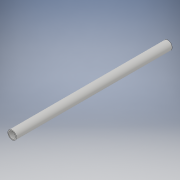
# Autodesk Inventor part: Prop Rod
Saved by Autodesk Inventor 2019 (Build 230136000, 136)
## iProperties
Created: 2019-10-06
Part Number: Prop Rod
Material: Generic
Document SubType Name: Modeling
Designer: robgr
Density: 1 g/cm^3
Appearance: Default
Author: robgr
Autodesk Inventor part; units mm, degrees
ref_plane "YZ Plane" through (0, 0, 0) normal (1, 0, 0) x (0, 1, 0)
ref_plane "XZ Plane" through (0, 0, 0) normal (0, 1, 0) x (-1, 0, 0)
sketch "Sketch1" plane through (0, 0, 0) normal (0, 0, 1) x (1, 0, 0)
  circle A0 centre (0, 0) radius 7.5
  circle A1 centre (0, 0) radius 6
  dimension "d0" = 15
  dimension "d1" = 12
  constraints: 2 centre point, 2 coincident
  measures "d0" diameter of A0
  measures "d1" diameter of A1
extrude "Extrusion1" add sketch "Sketch1" along normal blind 270
ref_plane "Work Plane1" through (0, 0, 135) normal (0, 0, 1) x (1, 0, 0)
body "Solid1"
